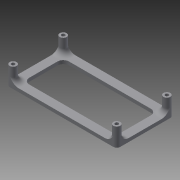
# Autodesk Inventor part: standoff
Saved by Autodesk Inventor 2013 (Build 170138000, 138)
## iProperties
Created: 2013-07-26
Part Number: standoff
Material: Generic
Document SubType Name: Modeling
Designer: employee
Density: 1 g/cm^3
Author: employee
Autodesk Inventor part; units mm, degrees
ref_plane "YZ Plane" through (0, 0, 0) normal (1, 0, 0) x (0, 1, 0)
ref_plane "XZ Plane" through (0, 0, 0) normal (0, 1, 0) x (-1, 0, 0)
ref_plane "XY Plane" through (0, 0, 0) normal (0, 0, 1) x (1, 0, 0)
sketch "Sketch1" plane through (0, 0, 0) normal (0, 0, 1) x (1, 0, 0)
  line L0 (0, 0) -> (101.6, 0)
  line L1 (101.6, 0) -> (101.6, 50.8)
  line L2 (101.6, 50.8) -> (0, 50.8)
  line L3 (0, 50.8) -> (0, 0)
  dimension "d0" = 50.8
  dimension "d2" = 101.6
  constraints: 8 end point, 2 parallel, 1 horizontal, 1 perpendicular
  measures "d0" distance of L0.end L1.end
  measures "d2" distance of L0.start L0.end
extrude "Extrusion1" add sketch "Sketch1" along normal blind 16
sketch "Sketch2" plane through (0, 0, 16) normal (0, 0, 1) x (1, 0, 0)
  line L0 (101.6, 0) -> (101.6, 50.8) projected
  line L1 (101.6, 50.8) -> (0, 50.8) projected
  line L2 (5.461, 47.3075) -> (96.139, 47.3075)
  line L3 (96.139, 47.3075) -> (96.139, 3.4925)
  line L4 (96.139, 3.4925) -> (5.461, 3.4925)
  line L5 (5.461, 3.4925) -> (5.461, 47.3075)
  point P0 (96.139, 25.4)
  point P1 (101.6, 25.4)
  point P2 (50.8, 47.3075)
  point P3 (50.8, 50.8)
  dimension "d5" = 43.815
  dimension "d7" = 90.678
  constraints: 8 end point, 4 midpoint, 2 parallel, 1 horizontal, 1 horizontal alignment, 1 perpendicular, 1 vertical alignment
  measures "d5" distance of L2.end L3.end
  measures "d7" distance of L2.start L2.end
hole "Hole1" at (5.461, 47.3075, 16) at (96.139, 47.3075, 16) at (96.139, 3.4925, 16) at (5.461, 3.4925, 16) direction (0, 0, -1) diameter 3 end through all clearance for "Socket Head Cap Screw" size "M3" standard "Ansi Metric M Profile"
sketch "Sketch3" plane through (0, 0, 16) normal (0, 0, 1) x (1, 0, 0)
  circle A0 centre (96.139, 3.4925) radius 1.5 projected
  circle A1 centre (5.461, 47.3075) radius 1.5 projected
  circle A2 centre (96.139, 47.3075) radius 1.5 projected
  circle A3 centre (5.461, 3.4925) radius 1.5 projected
  line L0 (0, 0) -> (101.6, 0) projected
  line L1 (101.6, 0) -> (101.6, 50.8) projected
  line L2 (101.6, 50.8) -> (0, 50.8) projected
  line L3 (0, 50.8) -> (0, 0) projected
  circle A4 centre (5.461, 3.4925) radius 3
  circle A5 centre (5.461, 47.3075) radius 3
  circle A6 centre (96.139, 47.3075) radius 3
  circle A7 centre (96.139, 3.4925) radius 3
  dimension "d15" = 6
  constraints: 4 centre point, 4 coincident, 3 equal radius
  measures "d15" diameter of A4
extrude "Extrusion2" cut sketch "Sketch3" against normal through all contours L3 L2 L1 L0
sketch "Sketch4" plane through (5.461, 3.4925, 0) normal (0, 0, -1) x (-1, 0, 0)
  circle A0 centre (0, 0) radius 3 projected
  circle A1 centre (-90.678, 0) radius 3 projected
  circle A2 centre (-90.678, 0) radius 1.5 projected
  circle A3 centre (0, 43.815) radius 1.5 projected
  circle A4 centre (0, 43.815) radius 3 projected
  circle A5 centre (-90.678, 43.815) radius 3 projected
  circle A6 centre (-90.678, 43.815) radius 1.5 projected
  circle A7 centre (0, 0) radius 1.5 projected
  circle A8 centre (0, 0) radius 3 projected
  line L0 (-90.678, 46.815) -> (0, 46.815)
  line L1 (-90.678, -3) -> (0, -3)
  line L2 (3, 0) -> (3, 43.815)
  line L3 (-93.678, 43.815) -> (-93.678, 0)
  circle A9 centre (-90.678, 43.815) radius 3 projected
  circle A10 centre (-90.678, 0) radius 3 projected
  point P0 (5.461, -3.4925)
  constraints: 10 point on circle, 8 end point, 7 tangent, 1 perpendicular
extrude "Extrusion3" add sketch "Sketch4" against normal blind 3 contours A0 L1 A1 L3 A5 L0 A4 L2
sketch "Sketch5" plane through (5.461, 3.4925, 3) normal (0, 0, 1) x (1, 0, 0)
  line L0 (90.678, 46.815) -> (0, 46.815) projected
  line L1 (93.678, 0) -> (93.678, 43.815) projected
  line L2 (4.5, 39.315) -> (86.178, 39.315)
  line L3 (86.178, 39.315) -> (86.178, 4.5)
  line L4 (86.178, 4.5) -> (4.5, 4.5)
  line L5 (4.5, 4.5) -> (4.5, 39.315)
  point P0 (-5.461, -3.4925)
  point P1 (86.178, 21.9075)
  point P2 (93.678, 21.9075)
  point P3 (45.339, 39.315)
  point P4 (45.339, 46.815)
  dimension "d21" = 7.5
  dimension "d22" = 7.5
  constraints: 8 end point, 4 midpoint, 2 parallel, 1 horizontal, 1 horizontal alignment, 1 perpendicular, 1 vertical alignment
  measures "d21" distance between parallel lines of L0 L2
  measures "d22" distance between parallel lines of L1 L3
extrude "Extrusion4" cut sketch "Sketch5" against normal through all
fillet "Fillet1" radius 5 6 edges at (5.461, 44.3075, 3) (7.5823, 49.4288, 3) (5.461, 6.4925, 3) (7.5823, 1.3712, 3) (94.0177, 5.6138, 3) (94.0177, 45.1862, 3)
fillet "Fillet2" radius 5 4 edges at (9.961, 7.9925, 1.6376) (9.961, 42.8075, 1.6376) (91.639, 42.8075, 1.6376) (91.639, 7.9925, 1.6376)
body "Solid1"
